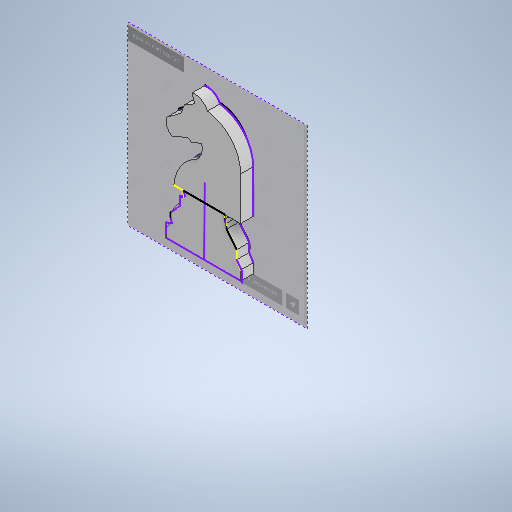
# Autodesk Inventor part: KINGHT 1.0
Saved by Autodesk Inventor 2025.1 (Build 291241000, 241)
## iProperties
Created: 2024-10-23
Part Number: KINGHT 1.0
Material: Genérico
Document SubType Name: Modeling
Designer: Octavio
Density: 1 g/cm^3
Appearance: Valor por defecto
Author: Octavio
Autodesk Inventor part; units mm, degrees
ref_plane "YZ Plane" through (0, 0, 0) normal (1, 0, 0) x (0, 1, 0)
ref_plane "XZ Plane" through (0, 0, 0) normal (0, 1, 0) x (-1, 0, 0)
ref_plane "XY Plane" through (0, 0, 0) normal (0, 0, 1) x (1, 0, 0)
sketch "Boceto1" plane through (0, 0, 0) normal (0, 0, 1) x (1, 0, 0)
  line L0 (-71.1055, 70.4875) -> (71.7516, 70.4875) construction
  line L1 (71.7516, 70.4875) -> (71.7516, -69.9887) construction
  line L2 (71.7516, -69.9887) -> (-71.1055, -69.9887) construction
  line L3 (-71.1055, -69.9887) -> (-71.1055, 70.4875) construction
  line L4 (-16.344, -18.0372) -> (15.0954, -18.0372)
  point P0 (0, 0)
  constraints: 2 end point, 1 horizontal, 2 other
sketch "Boceto2" plane through (0, 0, 0) normal (0, 0, 1) x (1, 0, 0)
  line L0 (-30.1866, -53.4632) -> (28.6068, -53.4632)
  line L1 (28.6068, -53.4632) -> (28.6068, -45.7841)
  line L2 (28.6068, -45.7841) -> (25.4871, -40.2647)
  line L3 (25.4871, -40.2647) -> (25.4871, -33.3055)
  line L4 (25.4871, -33.3055) -> (19.4878, -25.8663)
  line L5 (19.4878, -25.8663) -> (17.4099, -23.2897)
  line L6 (17.4099, -23.2897) -> (17.4099, -19.147)
  line L7 (17.4099, -19.147) -> (15.8731, -17.2414)
  line L8 (15.8731, -17.2414) -> (15.8731, -13.8176)
  line L9 (15.8731, -13.8176) -> (28.6068, -13.8176)
  line L10 (28.6068, -13.8176) -> (28.6068, 15.1601)
  line L11 (-30.1866, -53.4632) -> (-30.1866, -45.7841)
  line L12 (-30.1866, -45.7841) -> (-26.4512, -40.2647)
  line L13 (-26.4512, -40.2647) -> (-27.2401, -37.2121)
  line L14 (-27.2401, -37.2121) -> (-27.2401, -33.9857)
  line L15 (-27.2401, -33.9857) -> (-19.5651, -22.6451)
  line L16 (-19.5651, -22.6451) -> (-19.5651, -19.9512)
  line L17 (-19.5651, -19.9512) -> (-16.9146, -18.1942)
  line L18 (-16.9146, -18.1942) -> (-16.9146, -13.8176)
  line L19 (-16.9146, -13.8176) -> (-24.4978, -13.8176)
  arc A0 (-6.2899, 13.0619) -> (-24.4978, -13.8176) centre (7.8446, -16.1193) ccw
  arc A1 (-6.2899, 13.0619) -> (-2.4548, 26.1011) centre (-14.9411, 22.69) ccw
  line L20 (-2.4548, 26.1011) -> (-10.0959, 22.69)
  line L21 (-10.0959, 22.69) -> (-13.96, 24.3955)
  line L22 (-13.96, 24.3955) -> (-25.9619, 19.0376)
  arc A2 (-30.1866, 30.1701) -> (-25.9619, 19.0376) centre (-21.015, 27.2828) ccw
  line L23 (-30.1866, 30.1701) -> (-19.0004, 38.444)
  line L24 (-19.0004, 38.444) -> (-15.9019, 45.9592)
  line L25 (-15.9019, 45.9592) -> (-7.7883, 50.5452)
  line L26 (-7.7883, 50.5452) -> (-10.0959, 56.9512)
  arc A3 (2.199, 50.5452) -> (-10.0959, 56.9512) centre (-7.6346, 46.6736) ccw
  arc A4 (28.6068, 20.3485) -> (2.199, 50.5452) centre (-1.5881, 20.5877) ccw
  line L27 (28.6068, 20.3485) -> (28.6068, -13.8176)
  line L28 (-16.9146, -13.8176) -> (15.8731, -13.8176)
  point P0 (0, 0)
  constraints: 58 end point, 10 point on circle, 9 parallel, 5 centre point, 4 point on line, 3 perpendicular, 2 collinear, 1 horizontal, 1 vertical
extrude "Extrusión1" add sketch "Boceto2" along normal blind 10
sketch "Boceto3" plane through (0, 0, 10) normal (0, 0, 1) x (1, 0, 0)
  line L0 (-16.9146, -13.8176) -> (-16.9146, -18.1942) projected
  line L1 (15.8731, -17.2414) -> (15.8731, -13.8176) projected
  line L2 (-16.9146, -13.8176) -> (15.8731, -13.8176)
  line L3 (15.8731, -13.8176) -> (15.8731, -17.2414)
  line L4 (15.8731, -17.2414) -> (17.4099, -21.9355)
  line L5 (17.4099, -23.2897) -> (17.4099, -19.147) projected
  line L6 (17.4099, -21.9355) -> (17.4099, -23.2897)
  line L7 (17.4099, -23.2897) -> (18.0548, -23.9053)
  line L8 (25.4871, -40.2647) -> (25.4871, -33.3055) projected
  line L9 (29.7175, -53.186) -> (29.9979, -54.0424)
  line L10 (29.9979, -54.0424) -> (29.9979, -53.186)
  line L11 (29.9979, -53.186) -> (-30.6163, -53.186)
  line L12 (-30.6163, -53.186) -> (-30.6163, -42.5113)
  line L13 (-30.6163, -42.5113) -> (-26, -41)
  line L14 (-27.2401, -33.9857) -> (-27.2401, -37.2121) projected
  line L15 (-26, -41) -> (-27.2401, -37.2121)
  line L16 (-27.2401, -37.2121) -> (-27.2401, -33.9857)
  line L17 (-27.2401, -33.9857) -> (-19.7765, -26.1669)
  line L18 (-19.7765, -26.1669) -> (-19.7765, -18.6785)
  line L19 (-19.7765, -18.6785) -> (-15.3627, -17.2335)
  line L20 (-15.3627, -17.2335) -> (-16.9146, -13.8176)
  line L21 (0, 0) -> (-0.3092, -53.186)
  line L22 (29.7175, -53.186) -> (29.7175, -46)
  line L23 (28.6068, -45.7841) -> (25.4871, -40.2647) projected
  line L24 (29.7175, -46) -> (25.4871, -40.2647)
  line L25 (25.4871, -33.3055) -> (17.4099, -23.2897) projected
  line L26 (25.4871, -33.3055) -> (17.4099, -23.2897)
  line L27 (-24.4978, -13.8176) -> (-16.9146, -13.8176) projected
  line L28 (-16.9146, -13.8176) -> (15.8731, -13.8176)
  constraints: 42 end point, 6 parallel, 6 perpendicular, 2 collinear, 2 point on line, 1 horizontal, 1 midpoint, 1 vertical
